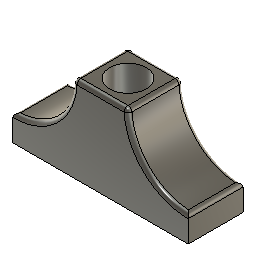
9mm_Belt_Clamp_2_Final_x2 v1 (Autodesk Fusion 360 design; units mm, degrees)
Autodesk Fusion 360 part; units mm, degrees
sketch "Sketch1" plane through (0, 0, 0) normal (0, 0, 1) x (1, 0, 0)
  line L0 (-11.2, 3.5) -> (11.2, 3.5)
  line L1 (11.2, 3.5) -> (11.2, -3.5)
  line L2 (11.2, -3.5) -> (-11.2, -3.5)
  line L3 (-11.2, -3.5) -> (-11.2, 3.5)
  line L4 (-11.2, 3.5) -> (11.2, -3.5) construction
  line L5 (11.2, 3.5) -> (-11.2, -3.5) construction
  circle A0 centre (0, 0) radius 1.6
  dimension "d1" = 22.4
  dimension "d2" = 7
  dimension "d3" = 3.2
  constraint horizontal L0
  constraint perpendicular L0 L1
  constraint parallel L0 L2
  constraint parallel L1 L3
  constraint coincident L4 A0.centre
  constraint coincident L5 A0.centre
  constraint coincident A0.centre origin
  measures "d1" distance of L1.end L2.end
  measures "d2" distance of L0.end L1.end
  measures "d3" diameter of A0
extrude "Extrude1" add sketch "Sketch1" along normal blind 11
sketch "Sketch2" plane through (0, 0, 11) normal (0, 0, 1) x (-1, 0, 0)
  circle A0 centre (0, 0) radius 1.6
  line L0 (11.2, 3.5) -> (-11.2, 3.5)
  line L1 (-11.2, 3.5) -> (-11.2, -3.5)
  line L2 (-11.2, -3.5) -> (11.2, -3.5)
  line L3 (11.2, -3.5) -> (11.2, 3.5)
  circle A1 centre (0, 0) radius 2.35
  dimension "d6" = 4.7
  constraint coincident A0.centre A1.centre
  measures "d6" diameter of A1
extrude "Extrude2" cut sketch "Sketch2" against normal blind 6 contours A1
sketch "Sketch3" plane through (0, -3.5, 0) normal (0, -1, 0) x (1, 0, 0)
  line L0 (-11.2, 0) -> (11.2, 0)
  line L1 (11.2, 0) -> (11.2, 11)
  line L2 (11.2, 11) -> (-11.2, 11)
  line L3 (-11.2, 11) -> (-11.2, 0)
  line L4 (0, 11) -> (-3.5, 11) construction
  arc A0 (-11.2, 3.3) -> (-3.5, 11) centre (-11.2, 11) ccw
  line L5 (0, 11) -> (3.5, 11) construction
  arc A1 (3.5, 11) -> (11.2, 3.3) centre (11.2, 11) ccw
  dimension "d9" = 3.5
  dimension "d10" = 3.5
  constraint midpoint L2 L4.start
  constraint parallel L2 L4
  constraint coincident L2.end L3.start
  constraint coincident L3 A0.start
  constraint parallel L2 L5
  constraint coincident L1.end L2.start
  constraint coincident L1 A1.end
  measures "d9" distance of L4.start L4.end
  measures "d10" distance of L4.start L5.end
extrude "Extrude3" cut sketch "Sketch3" against normal blind 7 contours L2 L3 A0 | L1 L2 A1
fillet "Fillet1" radius 0.5 10 edges at (11.2, 0, 3.3) (5.7553, 3.5, 5.5553) (5.7553, -3.5, 5.5553) (3.5, 0, 11) (0, 3.5, 11) (-3.5, 0, 11) (-5.7553, 3.5, 5.5553) (0, -3.5, 11) (-5.7553, -3.5, 5.5553) (-11.2, 0, 3.3)
